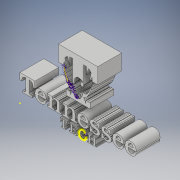
# Autodesk Inventor part: Main
Saved by Autodesk Inventor 2018 (Build 220112000, 112)
## iProperties
Created: 2017-12-08
Part Number: Main
Material: Generic
Document SubType Name: Modeling
Designer: Rus
Density: 1 g/cm^3
Appearance: Default
Author: Rus
Autodesk Inventor part; units mm, degrees
(part 1 of 3)
ref_plane "YZ Plane" through (0, 0, 0) normal (1, 0, 0) x (0, 1, 0)
ref_plane "XZ Plane" through (0, 0, 0) normal (0, 1, 0) x (-1, 0, 0)
ref_plane "XY Plane" through (0, 0, 0) normal (0, 0, 1) x (1, 0, 0)
sketch "Sketch1" plane through (0, 0, 0) normal (0, 0, 1) x (1, 0, 0)
  line L0 (63.7248, 41.0987) -> (64.7002, 37.0611)
  line L1 (64.7002, 37.0611) -> (64.5625, 36.9024)
  line L2 (64.5625, 36.9024) -> (63.8457, 36.2839)
  line L3 (63.8457, 36.2839) -> (63.0893, 35.88)
  line L4 (63.0893, 35.88) -> (62.9338, 35.8292)
  line L5 (62.9338, 35.8292) -> (61.9509, 40.717)
  line L6 (61.9509, 40.717) -> (61.0652, 35.7505)
  line L7 (61.0652, 35.7505) -> (60.894, 35.7889)
  line L8 (60.894, 35.7889) -> (60.0646, 36.1516)
  line L9 (60.0646, 36.1516) -> (59.2762, 36.7563)
  line L10 (59.2762, 36.7563) -> (59.1274, 36.9164)
  line L11 (59.1274, 36.9164) -> (60.1375, 41.0987)
  line L12 (60.1375, 41.0987) -> (58.1904, 38.2308)
  line L13 (58.1904, 38.2308) -> (58.0718, 38.4447)
  line L14 (58.0718, 38.4447) -> (57.5221, 39.6984)
  line L15 (57.5221, 39.6984) -> (57.0357, 41.2143)
  line L16 (57.0357, 41.2143) -> (56.9488, 41.5577)
  line L17 (56.9488, 41.5577) -> (55.9732, 44.7972)
  line L18 (55.9732, 44.7972) -> (55.9138, 44.5823)
  line L19 (55.9138, 44.5823) -> (55.6095, 43.9704)
  line L20 (55.6095, 43.9704) -> (55.1119, 43.5117)
  line L21 (55.1119, 43.5117) -> (54.5249, 43.3598)
  line L22 (54.5249, 43.3598) -> (53.8897, 43.4538)
  line L23 (53.8897, 43.4538) -> (53.2501, 43.7363)
  line L24 (53.2501, 43.7363) -> (52.6479, 44.1442)
  line L25 (52.6479, 44.1442) -> (52.1272, 44.6181)
  line L26 (52.1272, 44.6181) -> (51.8185, 44.971)
  line L27 (51.8185, 44.971) -> (51.7301, 45.0977)
  line L28 (51.7301, 45.0977) -> (51.1693, 45.9052)
  line L29 (51.1693, 45.9052) -> (49.7197, 48.4838)
  line L30 (49.7197, 48.4838) -> (48.2547, 51.9024)
  line L31 (48.2547, 51.9024) -> (47.3149, 55.134)
  line L32 (47.3149, 55.134) -> (46.9331, 57.2478)
  line L33 (46.9331, 57.2478) -> (46.8823, 57.9562)
  line L34 (46.8823, 57.9562) -> (46.8754, 57.8239)
  line L35 (46.8754, 57.8239) -> (46.845, 56.435)
  line L36 (46.845, 56.435) -> (46.8465, 56.2889)
  line L37 (46.8465, 56.2889) -> (46.8478, 55.5681)
  line L38 (46.8478, 55.5681) -> (47.147, 53.4045)
  line L39 (47.147, 53.4045) -> (48.0451, 49.9608)
  line L40 (48.0451, 49.9608) -> (49.5653, 46.2471)
  line L41 (49.5653, 46.2471) -> (51.1211, 43.4261)
  line L42 (51.1211, 43.4261) -> (51.7301, 42.5483)
  line L43 (51.7301, 42.5483) -> (51.8114, 42.431)
  line L44 (51.8114, 42.431) -> (52.0718, 42.0868)
  line L45 (52.0718, 42.0868) -> (52.528, 41.5369)
  line L46 (52.528, 41.5369) -> (53.0642, 40.9608)
  line L47 (53.0642, 40.9608) -> (53.6496, 40.4178)
  line L48 (53.6496, 40.4178) -> (54.2534, 39.973)
  line L49 (54.2534, 39.973) -> (54.8432, 39.686)
  line L50 (54.8432, 39.686) -> (55.3862, 39.6202)
  line L51 (55.3862, 39.6202) -> (55.7611, 39.7538)
  line L52 (55.7611, 39.7538) -> (55.8518, 39.8351)
  line L53 (55.8518, 39.8351) -> (55.8381, 39.7386)
  line L54 (55.8381, 39.7386) -> (55.5034, 38.7919)
  line L55 (55.5034, 38.7919) -> (55.4579, 38.7022)
  line L56 (55.4579, 38.7022) -> (53.5111, 34.8875)
  line L57 (53.5111, 34.8875) -> (53.5111, 38.0188)
  line L58 (53.5111, 38.0188) -> (53.4367, 38.0074)
  line L59 (53.4367, 38.0074) -> (52.6454, 37.9068)
  line L60 (52.6454, 37.9068) -> (52.5614, 37.8986)
  line L61 (52.5614, 37.8986) -> (52.3178, 37.875)
  line L62 (52.3178, 37.875) -> (50.9673, 37.7938)
  line L63 (50.9673, 37.7938) -> (49.567, 37.7592)
  line L64 (49.567, 37.7592) -> (49.1014, 37.7592)
  line L65 (49.1014, 37.7592) -> (49.1014, 32.2513)
  line L66 (49.1014, 32.2513) -> (74.6006, 32.2513)
  line L67 (74.6006, 32.2513) -> (74.6006, 37.7595)
  line L68 (74.6006, 37.7595) -> (74.1252, 37.7704)
  line L69 (74.1252, 37.7704) -> (72.1808, 37.841)
  line L70 (72.1808, 37.841) -> (70.8138, 37.9317)
  line L71 (70.8138, 37.9317) -> (70.6278, 37.9523)
  line L72 (70.6278, 37.9523) -> (70.5933, 37.9566)
  line L73 (70.5933, 37.9566) -> (70.2641, 37.9952)
  line L74 (70.2641, 37.9952) -> (70.2323, 37.9993)
  line L75 (70.2323, 37.9993) -> (70.2323, 34.8875)
  line L76 (70.2323, 34.8875) -> (68.2214, 38.8246)
  line L77 (68.2214, 38.8246) -> (68.1802, 38.9059)
  line L78 (68.1802, 38.9059) -> (67.9361, 39.6747)
  line L79 (67.9361, 39.6747) -> (67.9236, 39.7672)
  line L80 (67.9236, 39.7672) -> (68.0189, 39.6996)
  line L81 (68.0189, 39.6996) -> (68.3935, 39.6143)
  line L82 (68.3935, 39.6143) -> (68.9323, 39.7175)
  line L83 (68.9323, 39.7175) -> (69.5098, 40.0208)
  line L84 (69.5098, 40.0208) -> (70.0981, 40.4687)
  line L85 (70.0981, 40.4687) -> (70.6662, 41.0034)
  line L86 (70.6662, 41.0034) -> (71.1853, 41.5655)
  line L87 (71.1853, 41.5655) -> (71.6262, 42.1005)
  line L88 (71.6262, 42.1005) -> (71.88, 42.434)
  line L89 (71.88, 42.434) -> (71.9597, 42.5483)
  line L90 (71.9597, 42.5483) -> (72.5675, 43.4261)
  line L91 (72.5675, 43.4261) -> (74.1218, 46.2471)
  line L92 (74.1218, 46.2471) -> (75.642, 49.9608)
  line L93 (75.642, 49.9608) -> (76.5419, 53.4045)
  line L94 (76.5419, 53.4045) -> (76.8406, 55.5681)
  line L95 (76.8406, 55.5681) -> (76.8434, 56.2889)
  line L96 (76.8434, 56.2889) -> (76.8434, 56.435)
  line L97 (76.8434, 56.435) -> (76.8132, 57.8239)
  line L98 (76.8132, 57.8239) -> (76.8078, 57.9562)
  line L99 (76.8078, 57.9562) -> (76.7552, 57.2463)
  line L100 (76.7552, 57.2463) -> (76.3735, 55.134)
  line L101 (76.3735, 55.134) -> (75.4337, 51.9024)
  line L102 (75.4337, 51.9024) -> (73.9676, 48.4838)
  line L103 (73.9676, 48.4838) -> (72.519, 45.9039)
  line L104 (72.519, 45.9039) -> (71.9597, 45.0977)
  line L105 (71.9597, 45.0977) -> (71.8703, 44.971)
  line L106 (71.8703, 44.971) -> (71.5617, 44.6181)
  line L107 (71.5617, 44.6181) -> (71.0408, 44.1442)
  line L108 (71.0408, 44.1442) -> (70.4385, 43.7363)
  line L109 (70.4385, 43.7363) -> (69.7989, 43.4538)
  line L110 (69.7989, 43.4538) -> (69.1639, 43.3598)
  line L111 (69.1639, 43.3598) -> (68.5754, 43.5117)
  line L112 (68.5754, 43.5117) -> (68.0791, 43.9704)
  line L113 (68.0791, 43.9704) -> (67.7746, 44.5823)
  line L114 (67.7746, 44.5823) -> (67.7167, 44.7972)
  line L115 (67.7167, 44.7972) -> (66.74, 41.5577)
  line L116 (66.74, 41.5577) -> (66.657, 41.2323)
  line L117 (66.657, 41.2323) -> (66.2008, 39.7881)
  line L118 (66.2008, 39.7881) -> (65.6869, 38.578)
  line L119 (65.6869, 38.578) -> (65.5767, 38.3703)
  line L120 (65.5767, 38.3703) -> (63.7248, 41.0987)
  line L121 (82.8011, 75.2394) -> (82.8011, 58.6456)
  line L122 (82.8011, 58.6456) -> (76.9705, 58.6456)
  line L123 (76.9705, 58.6456) -> (76.9705, 59.5536)
  line L124 (76.9705, 59.5536) -> (76.7432, 62.0052)
  line L125 (76.7432, 62.0052) -> (76.6974, 62.2752)
  line L126 (76.6974, 62.2752) -> (73.8313, 57.2978)
  line L127 (73.8313, 57.2978) -> (75.8254, 65.5592)
  line L128 (75.8254, 65.5592) -> (75.6723, 65.9148)
  line L129 (75.6723, 65.9148) -> (74.6885, 67.3796)
  line L130 (74.6885, 67.3796) -> (73.3972, 68.4558)
  line L131 (73.3972, 68.4558) -> (73.0924, 68.6156)
  line L132 (73.0924, 68.6156) -> (70.874, 61.7462)
  line L133 (70.874, 61.7462) -> (70.7833, 69.3639)
  line L134 (70.7833, 69.3639) -> (70.5542, 69.4037)
  line L135 (70.5542, 69.4037) -> (67.9857, 69.546)
  line L136 (67.9857, 69.546) -> (67.7002, 69.5346)
  line L137 (67.7002, 69.5346) -> (67.7117, 50.8236)
  line L138 (67.7117, 50.8236) -> (67.7117, 50.544)
  line L139 (67.7117, 50.544) -> (67.4744, 49.7022)
  line L140 (67.4744, 49.7022) -> (66.8609, 48.954)
  line L141 (66.8609, 48.954) -> (66.023, 48.6754)
  line L142 (66.023, 48.6754) -> (65.3008, 48.8355)
  line L143 (65.3008, 48.8355) -> (65.1109, 48.9623)
  line L144 (65.1109, 48.9623) -> (64.9321, 49.0822)
  line L145 (64.9321, 49.0822) -> (64.5267, 49.6308)
  line L146 (64.5267, 49.6308) -> (64.2924, 50.529)
  line L147 (64.2924, 50.529) -> (64.4718, 51.4815)
  line L148 (64.4718, 51.4815) -> (64.928, 52.1525)
  line L149 (64.928, 52.1525) -> (65.132, 52.3067)
  line L150 (65.132, 52.3067) -> (66.0855, 52.4872)
  line L151 (66.0855, 52.4872) -> (66.6036, 52.1895)
  line L152 (66.6036, 52.1895) -> (66.6369, 52.432)
  line L153 (66.6369, 52.432) -> (66.5816, 53.1803)
  line L154 (66.5816, 53.1803) -> (66.2235, 53.8128)
  line L155 (66.2235, 53.8128) -> (65.5952, 54.1575)
  line L156 (65.5952, 54.1575) -> (64.9693, 54.2719)
  line L157 (64.9693, 54.2719) -> (64.7598, 54.2788)
  line L158 (64.7598, 54.2788) -> (64.4337, 54.4825)
  line L159 (64.4337, 54.4825) -> (63.3298, 54.8895)
  line L160 (63.3298, 54.8895) -> (61.9572, 54.9707)
  line L161 (61.9572, 54.9707) -> (60.6991, 54.592)
  line L162 (60.6991, 54.592) -> (59.6089, 53.8215)
  line L163 (59.6089, 53.8215) -> (58.7472, 52.7319)
  line L164 (58.7472, 52.7319) -> (58.1687, 51.3896)
  line L165 (58.1687, 51.3896) -> (57.9301, 49.8656)
  line L166 (57.9301, 49.8656) -> (57.9988, 48.6253)
  line L167 (57.9988, 48.6253) -> (58.0882, 48.2255)
  line L168 (58.0882, 48.2255) -> (58.1258, 48.0576)
  line L169 (58.1258, 48.0576) -> (58.1006, 47.4831)
  line L170 (58.1006, 47.4831) -> (57.7932, 47.1882)
  line L171 (57.7932, 47.1882) -> (57.6898, 47.1605)
  line L172 (57.6898, 47.1605) -> (57.5163, 47.1151)
  line L173 (57.5163, 47.1151) -> (56.9388, 47.1852)
  line L174 (56.9388, 47.1852) -> (56.4031, 47.6234)
  line L175 (56.4031, 47.6234) -> (56.0821, 48.3415)
  line L176 (56.0821, 48.3415) -> (55.976, 48.9892)
  line L177 (55.976, 48.9892) -> (55.976, 49.2044)
  line L178 (55.976, 49.2044) -> (55.9897, 69.5355)
  line L179 (55.9897, 69.5355) -> (55.703, 69.547)
  line L180 (55.703, 69.547) -> (53.1343, 69.4047)
  line L181 (53.1343, 69.4047) -> (52.9072, 69.3649)
  line L182 (52.9072, 69.3649) -> (52.816, 61.7471)
  line L183 (52.816, 61.7471) -> (50.5976, 68.6166)
  line L184 (50.5976, 68.6166) -> (50.2917, 68.4568)
  line L185 (50.2917, 68.4568) -> (49.0014, 67.3791)
  line L186 (49.0014, 67.3791) -> (48.0162, 65.9145)
  line L187 (48.0162, 65.9145) -> (47.8648, 65.5602)
  line L188 (47.8648, 65.5602) -> (49.8574, 57.2988)
  line L189 (49.8574, 57.2988) -> (47.0063, 62.2529)
  line L190 (47.0063, 62.2529) -> (46.9593, 61.9841)
  line L191 (46.9593, 61.9841) -> (46.7307, 59.4815)
  line L192 (46.7307, 59.4815) -> (46.7307, 58.6466)
  line L193 (46.7307, 58.6466) -> (40.9636, 58.6466)
  line L194 (40.9636, 58.6466) -> (40.9636, 75.2394)
  line L195 (40.9636, 75.2394) -> (82.8011, 75.2394)
  line L196 (6.1983, 26.6612) -> (5.8648, 26.6612)
  line L197 (5.8648, 26.6612) -> (5.4238, 26.6612)
  line L198 (5.4238, 26.6612) -> (4.1051, 26.3565)
  line L199 (4.1051, 26.3565) -> (3.0565, 25.6467)
  line L200 (3.0565, 25.6467) -> (2.9022, 25.4442)
  line L201 (2.9022, 25.4442) -> (2.7478, 25.2415)
  line L202 (2.7478, 25.2415) -> (2.198, 23.8497)
  line L203 (2.198, 23.8497) -> (1.9444, 21.9535)
  line L204 (1.9444, 21.9535) -> (1.9389, 21.4988)
  line L205 (1.9389, 21.4988) -> (0, 21.4988)
  line L206 (0, 21.4988) -> (0, 28.5255)
  line L207 (0, 28.5255) -> (15.9768, 28.5255)
  line L208 (15.9768, 28.5255) -> (15.9768, 21.4991)
  line L209 (15.9768, 21.4991) -> (14.0379, 21.4991)
  line L210 (14.0379, 21.4991) -> (14.0338, 21.9483)
  line L211 (14.0338, 21.9483) -> (13.7871, 23.828)
  line L212 (13.7871, 23.828) -> (13.2414, 25.2212)
  line L213 (13.2414, 25.2212) -> (13.0871, 25.4265)
  line L214 (13.0871, 25.4265) -> (12.9327, 25.6333)
  line L215 (12.9327, 25.6333) -> (11.8854, 26.3526)
  line L216 (11.8854, 26.3526) -> (10.5736, 26.6612)
  line L217 (10.5736, 26.6612) -> (10.1367, 26.6612)
  line L218 (10.1367, 26.6612) -> (9.766, 26.6612)
  line L219 (9.766, 26.6612) -> (9.766, 15.0554)
  line L220 (9.766, 15.0554) -> (9.766, 14.8473)
  line L221 (9.766, 14.8473) -> (9.8349, 14.2189)
  line L222 (9.8349, 14.2189) -> (9.9975, 13.8041)
  line L223 (9.9975, 13.8041) -> (10.0444, 13.7587)
  line L224 (10.0444, 13.7587) -> (10.0898, 13.7132)
  line L225 (10.0898, 13.7132) -> (10.5363, 13.5547)
  line L226 (10.5363, 13.5547) -> (11.2267, 13.4872)
  line L227 (11.2267, 13.4872) -> (11.4582, 13.4872)
  line L228 (11.4582, 13.4872) -> (12.9024, 13.4872)
  line L229 (12.9024, 13.4872) -> (12.9024, 11.5607)
  line L230 (12.9024, 11.5607) -> (3.0618, 11.5607)
  line L231 (3.0618, 11.5607) -> (3.0618, 13.4872)
  line L232 (3.0618, 13.4872) -> (4.5308, 13.4872)
  line L233 (4.5308, 13.4872) -> (4.7582, 13.4872)
  line L234 (4.7582, 13.4872) -> (5.4417, 13.5533)
  line L235 (5.4417, 13.5533) -> (5.8813, 13.7077)
  line L236 (5.8813, 13.7077) -> (5.9268, 13.7518)
  line L237 (5.9268, 13.7518) -> (5.9709, 13.7973)
  line L238 (5.9709, 13.7973) -> (6.1293, 14.2121)
  line L239 (6.1293, 14.2121) -> (6.1983, 14.8446)
  line L240 (6.1983, 14.8446) -> (6.1983, 15.0554)
  line L241 (6.1983, 15.0554) -> (6.1983, 26.6612)
  line L242 (24.6021, 19.0679) -> (24.5828, 19.3435)
  line L243 (24.5828, 19.3435) -> (24.3775, 20.4997)
  line L244 (24.3775, 20.4997) -> (24.022, 21.3596)
  line L245 (24.022, 21.3596) -> (23.9282, 21.4864)
  line L246 (23.9282, 21.4864) -> (23.8345, 21.6145)
  line L247 (23.8345, 21.6145) -> (23.2351, 22.0624)
  line L248 (23.2351, 22.0624) -> (22.5185, 22.2526)
  line L249 (22.5185, 22.2526) -> (22.2801, 22.2526)
  line L250 (22.2801, 22.2526) -> (22.0279, 22.2526)
  line L251 (22.0279, 22.2526) -> (21.2728, 22.0514)
  line L252 (21.2728, 22.0514) -> (20.5879, 21.5787)
  line L253 (20.5879, 21.5787) -> (20.4721, 21.4437)
  line L254 (20.4721, 21.4437) -> (20.355, 21.31)
  line L255 (20.355, 21.31) -> (19.892, 20.4459)
  line L256 (19.892, 20.4459) -> (19.5888, 19.3298)
  line L257 (19.5888, 19.3298) -> (19.5516, 19.0679)
  line L258 (19.5516, 19.0679) -> (24.6021, 19.0679)
  line L259 (25.7492, 15.8331) -> (27.8727, 15.8331)
  line L260 (27.8727, 15.8331) -> (27.8273, 15.4679)
  line L261 (27.8273, 15.4679) -> (27.2972, 13.8693)
  line L262 (27.2972, 13.8693) -> (26.3617, 12.5807)
  line L263 (26.3617, 12.5807) -> (26.1135, 12.3698)
  line L264 (26.1135, 12.3698) -> (25.8657, 12.1589)
  line L265 (25.8657, 12.1589) -> (24.4174, 11.4214)
  line L266 (24.4174, 11.4214) -> (22.8327, 11.1042)
  line L267 (22.8327, 11.1042) -> (22.3049, 11.1042)
  line L268 (22.3049, 11.1042) -> (21.9618, 11.1042)
  line L269 (21.9618, 11.1042) -> (20.9338, 11.2145)
  line L270 (20.9338, 11.2145) -> (19.7087, 11.541)
  line L271 (19.7087, 11.541) -> (18.6297, 12.0868)
  line L272 (18.6297, 12.0868) -> (17.909, 12.638)
  line L273 (17.909, 12.638) -> (17.6995, 12.8502)
  line L274 (17.6995, 12.8502) -> (17.4887, 13.0652)
  line L275 (17.4887, 13.0652) -> (16.9485, 13.7983)
  line L276 (16.9485, 13.7983) -> (16.4124, 14.8925)
  line L277 (16.4124, 14.8925) -> (16.09, 16.1355)
  line L278 (16.09, 16.1355) -> (15.9839, 17.1772)
  line L279 (15.9839, 17.1772) -> (15.9839, 17.5245)
  line L280 (15.9839, 17.5245) -> (15.9839, 17.869)
  line L281 (15.9839, 17.869) -> (16.0914, 18.8998)
  line L282 (16.0914, 18.8998) -> (16.4166, 20.1345)
  line L283 (16.4166, 20.1345) -> (16.9581, 21.2301)
  line L284 (16.9581, 21.2301) -> (17.5066, 21.9687)
  line L285 (17.5066, 21.9687) -> (17.7188, 22.185)
  line L286 (17.7188, 22.185) -> (17.9297, 22.4014)
  line L287 (17.9297, 22.4014) -> (18.6545, 22.9609)
  line L288 (18.6545, 22.9609) -> (19.7321, 23.5134)
  line L289 (19.7321, 23.5134) -> (20.9476, 23.8456)
  line L290 (20.9476, 23.8456) -> (21.9645, 23.9558)
  line L291 (21.9645, 23.9558) -> (22.3049, 23.9558)
  line L292 (22.3049, 23.9558) -> (22.6274, 23.9558)
  line L293 (22.6274, 23.9558) -> (23.5989, 23.8497)
  line L294 (23.5989, 23.8497) -> (24.7303, 23.53)
  line L295 (24.7303, 23.53) -> (25.699, 22.9953)
  line L296 (25.699, 22.9953) -> (26.3273, 22.4551)
  line L297 (26.3273, 22.4551) -> (26.5039, 22.247)
  line L298 (26.5039, 22.247) -> (26.6857, 22.0307)
  line L299 (26.6857, 22.0307) -> (27.1351, 21.2948)
  line L300 (27.1351, 21.2948) -> (27.5856, 20.1496)
  line L301 (27.5856, 20.1496) -> (27.8569, 18.8102)
  line L302 (27.8569, 18.8102) -> (27.9479, 17.6601)
  line L303 (27.9479, 17.6601) -> (27.9479, 17.2771)
  line L304 (27.9479, 17.2771) -> (19.4279, 17.2771)
  line L305 (19.4279, 17.2771) -> (19.4389, 16.9409)
  line L306 (19.4389, 16.9409) -> (19.6789, 15.494)
  line L307 (19.6789, 15.494) -> (20.1544, 14.3682)
  line L308 (20.1544, 14.3682) -> (20.2853, 14.1904)
  line L309 (20.2853, 14.1904) -> (20.4162, 14.014)
  line L310 (20.4162, 14.014) -> (21.228, 13.3954)
  line L311 (21.228, 13.3954) -> (22.1747, 13.1294)
  line L312 (22.1747, 13.1294) -> (22.4902, 13.1294)
  line L313 (22.4902, 13.1294) -> (22.8086, 13.1294)
  line L314 (22.8086, 13.1294) -> (23.7677, 13.2865)
  line L315 (23.7677, 13.2865) -> (24.5684, 13.6489)
  line L316 (24.5684, 13.6489) -> (24.6937, 13.7522)
  line L317 (24.6937, 13.7522) -> (24.8178, 13.8569)
  line L318 (24.8178, 13.8569) -> (25.3304, 14.5846)
  line L319 (25.3304, 14.5846) -> (25.6969, 15.5906)
  line L320 (25.6969, 15.5906) -> (25.7492, 15.8331)
  line L321 (28.9885, 11.5604) -> (28.9885, 13.2512)
  line L322 (28.9885, 13.2512) -> (29.829, 13.2512)
  line L323 (29.829, 13.2512) -> (30.0081, 13.2512)
  line L324 (30.0081, 13.2512) -> (30.5471, 13.3201)
  line L325 (30.5471, 13.3201) -> (30.9288, 13.4786)
  line L326 (30.9288, 13.4786) -> (30.9768, 13.5227)
  line L327 (30.9768, 13.5227) -> (31.0238, 13.5681)
  line L328 (31.0238, 13.5681) -> (31.1892, 13.9719)
  line L329 (31.1892, 13.9719) -> (31.2608, 14.5714)
  line L330 (31.2608, 14.5714) -> (31.2608, 14.7698)
  line L331 (31.2608, 14.7698) -> (31.2608, 20.2889)
  line L332 (31.2608, 20.2889) -> (31.2608, 20.4887)
  line L333 (31.2608, 20.4887) -> (31.1892, 21.0881)
  line L334 (31.1892, 21.0881) -> (31.0238, 21.4864)
  line L335 (31.0238, 21.4864) -> (30.9768, 21.5305)
  line L336 (30.9768, 21.5305) -> (30.9288, 21.5746)
  line L337 (30.9288, 21.5746) -> (30.5471, 21.7303)
  line L338 (30.5471, 21.7303) -> (30.0081, 21.7965)
  line L339 (30.0081, 21.7965) -> (29.829, 21.7965)
  line L340 (29.829, 21.7965) -> (28.9885, 21.7965)
  line L341 (28.9885, 21.7965) -> (28.9885, 23.4997)
  line L342 (28.9885, 23.4997) -> (34.3228, 23.4997)
  line L343 (34.3228, 23.4997) -> (34.3228, 21.401)
  line L344 (34.3228, 21.401) -> (34.4869, 21.6077)
  line L345 (34.4869, 21.6077) -> (36.1793, 23.1511)
  line L346 (36.1793, 23.1511) -> (36.354, 23.2531)
  line L347 (36.354, 23.2531) -> (36.5278, 23.3564)
  line L348 (36.5278, 23.3564) -> (37.9842, 23.8704)
  line L349 (37.9842, 23.8704) -> (38.4709, 23.8704)
  line L350 (38.4709, 23.8704) -> (38.9131, 23.8704)
  line L351 (38.9131, 23.8704) -> (40.2428, 23.6182)
  line L352 (40.2428, 23.6182) -> (41.2847, 23.0271)
  line L353 (41.2847, 23.0271) -> (41.4348, 22.8576)
  line L354 (41.4348, 22.8576) -> (41.5852, 22.6894)
  line L355 (41.5852, 22.6894) -> (42.1099, 21.5057)
  line L356 (42.1099, 21.5057) -> (42.3362, 19.983)
  line L357 (42.3362, 19.983) -> (42.3362, 19.4745)
  line L358 (42.3362, 19.4745) -> (42.3362, 14.7699)
  line L359 (42.3362, 14.7699) -> (42.3362, 14.5714)
  line L360 (42.3362, 14.5714) -> (42.4079, 13.972)
  line L361 (42.4079, 13.972) -> (42.577, 13.5682)
  line L362 (42.577, 13.5682) -> (42.6255, 13.5227)
  line L363 (42.6255, 13.5227) -> (42.6738, 13.4786)
  line L364 (42.6738, 13.4786) -> (43.0596, 13.3202)
  line L365 (43.0596, 13.3202) -> (43.5999, 13.2512)
  line L366 (43.5999, 13.2512) -> (43.7805, 13.2512)
  line L367 (43.7805, 13.2512) -> (44.5216, 13.2512)
  line L368 (44.5216, 13.2512) -> (44.5216, 11.5604)
  line L369 (44.5216, 11.5604) -> (37.3352, 11.5604)
  line L370 (37.3352, 11.5604) -> (37.3352, 13.2512)
  line L371 (37.3352, 13.2512) -> (37.8424, 13.2512)
  line L372 (37.8424, 13.2512) -> (38.0213, 13.2512)
  line L373 (38.0213, 13.2512) -> (38.5618, 13.3201)
  line L374 (38.5618, 13.3201) -> (38.9473, 13.4786)
  line L375 (38.9473, 13.4786) -> (38.9956, 13.5227)
  line L376 (38.9956, 13.5227) -> (39.0441, 13.5681)
  line L377 (39.0441, 13.5681) -> (39.2133, 13.9719)
  line L378 (39.2133, 13.9719) -> (39.2864, 14.5714)
  line L379 (39.2864, 14.5714) -> (39.2864, 14.7698)
  line L380 (39.2864, 14.7698) -> (39.2864, 19.4744)
  line L381 (39.2864, 19.4744) -> (39.2864, 19.7583)
  line L382 (39.2864, 19.7583) -> (39.1765, 20.6072)
  line L383 (39.1765, 20.6072) -> (38.9212, 21.27)
  line L384 (38.9212, 21.27) -> (38.8483, 21.3637)
  line L385 (38.8483, 21.3637) -> (38.7739, 21.4588)
  line L386 (38.7739, 21.4588) -> (38.2681, 21.7909)
  line L387 (38.2681, 21.7909) -> (37.623, 21.9315)
  line L388 (37.623, 21.9315) -> (37.4096, 21.9315)
  line L389 (37.4096, 21.9315) -> (37.0886, 21.9315)
  line L390 (37.0886, 21.9315) -> (36.1279, 21.66)
  line L391 (36.1279, 21.66) -> (35.2872, 21.0275)
  line L392 (35.2872, 21.0275) -> (35.1495, 20.8456)
  line L393 (35.1495, 20.8456) -> (35.0119, 20.6651)
  line L394 (35.0119, 20.6651) -> (34.5295, 19.5557)
  line L395 (34.5295, 19.5557) -> (34.3228, 18.2824)
  line L396 (34.3228, 18.2824) -> (34.3228, 17.8566)
  line L397 (34.3228, 17.8566) -> (34.3228, 14.7698)
  line L398 (34.3228, 14.7698) -> (34.3228, 14.5714)
  line L399 (34.3228, 14.5714) -> (34.3944, 13.9719)
  line L400 (34.3944, 13.9719) -> (34.5641, 13.5681)
  line L401 (34.5641, 13.5681) -> (34.6121, 13.5227)
  line L402 (34.6121, 13.5227) -> (34.6603, 13.4786)
  line L403 (34.6603, 13.4786) -> (35.0464, 13.3201)
  line L404 (35.0464, 13.3201) -> (35.5864, 13.2512)
  line L405 (35.5864, 13.2512) -> (35.767, 13.2512)
  line L406 (35.767, 13.2512) -> (36.274, 13.2512)
  line L407 (36.274, 13.2512) -> (36.274, 11.5604)
  line L408 (36.274, 11.5604) -> (28.9885, 11.5604)
  line L409 (45.3182, 11.5604) -> (45.3182, 13.2512)
  line L410 (45.3182, 13.2512) -> (46.1574, 13.2512)
  line L411 (46.1574, 13.2512) -> (46.3367, 13.2512)
  line L412 (46.3367, 13.2512) -> (46.8767, 13.3201)
  line L413 (46.8767, 13.3201) -> (47.2585, 13.4786)
  line L414 (47.2585, 13.4786) -> (47.3067, 13.5227)
  line L415 (47.3067, 13.5227) -> (47.3535, 13.5681)
  line L416 (47.3535, 13.5681) -> (47.5188, 13.9719)
  line L417 (47.5188, 13.9719) -> (47.5905, 14.5714)
  line L418 (47.5905, 14.5714) -> (47.5905, 14.7698)
  line L419 (47.5905, 14.7698) -> (47.5905, 20.2889)
  line L420 (47.5905, 20.2889) -> (47.5905, 20.4887)
  line L421 (47.5905, 20.4887) -> (47.5188, 21.0881)
  line L422 (47.5188, 21.0881) -> (47.3535, 21.4864)
  line L423 (47.3535, 21.4864) -> (47.3068, 21.5305)
  line L424 (47.3068, 21.5305) -> (47.2585, 21.5746)
  line L425 (47.2585, 21.5746) -> (46.8767, 21.7303)
  line L426 (46.8767, 21.7303) -> (46.3367, 21.7965)
  line L427 (46.3367, 21.7965) -> (46.1574, 21.7965)
  line L428 (46.1574, 21.7965) -> (45.3182, 21.7965)
  line L429 (45.3182, 21.7965) -> (45.3182, 23.4997)
  line L430 (45.3182, 23.4997) -> (50.6525, 23.4997)
  line L431 (50.6525, 23.4997) -> (50.6525, 21.401)
  line L432 (50.6525, 21.401) -> (50.8165, 21.6077)
  line L433 (50.8165, 21.6077) -> (52.5089, 23.1511)
  line L434 (52.5089, 23.1511) -> (52.6839, 23.2531)
  line L435 (52.6839, 23.2531) -> (52.8574, 23.3564)
  line L436 (52.8574, 23.3564) -> (54.3141, 23.8705)
  line L437 (54.3141, 23.8705) -> (54.8005, 23.8705)
  line L438 (54.8005, 23.8705) -> (55.243, 23.8705)
  line L439 (55.243, 23.8705) -> (56.5711, 23.6183)
  line L440 (56.5711, 23.6183) -> (57.6133, 23.0271)
  line L441 (57.6133, 23.0271) -> (57.7632, 22.8577)
  line L442 (57.7632, 22.8577) -> (57.9135, 22.6895)
  line L443 (57.9135, 22.6895) -> (58.4398, 21.5058)
  line L444 (58.4398, 21.5058) -> (58.6659, 19.983)
  line L445 (58.6659, 19.983) -> (58.6659, 19.4746)
  line L446 (58.6659, 19.4746) -> (58.6659, 14.7699)
  line L447 (58.6659, 14.7699) -> (58.6659, 14.5715)
  line L448 (58.6659, 14.5715) -> (58.7375, 13.9721)
  line L449 (58.7375, 13.9721) -> (58.9069, 13.5683)
  line L450 (58.9069, 13.5683) -> (58.9552, 13.5228)
  line L451 (58.9552, 13.5228) -> (59.0034, 13.4787)
  line L452 (59.0034, 13.4787) -> (59.388, 13.3202)
  line L453 (59.388, 13.3202) -> (59.9295, 13.2513)
  line L454 (59.9295, 13.2513) -> (60.1101, 13.2513)
  line L455 (60.1101, 13.2513) -> (60.8501, 13.2513)
  line L456 (60.8501, 13.2513) -> (60.8501, 11.5604)
  line L457 (60.8501, 11.5604) -> (53.6649, 11.5604)
  line L458 (53.6649, 11.5604) -> (53.6649, 13.2513)
  line L459 (53.6649, 13.2513) -> (54.1709, 13.2513)
  line L460 (54.1709, 13.2513) -> (54.35, 13.2513)
  line L461 (54.35, 13.2513) -> (54.8915, 13.3202)
  line L462 (54.8915, 13.3202) -> (55.2771, 13.4787)
  line L463 (55.2771, 13.4787) -> (55.3256, 13.5228)
  line L464 (55.3256, 13.5228) -> (55.3738, 13.5682)
  line L465 (55.3738, 13.5682) -> (55.5433, 13.972)
  line L466 (55.5433, 13.972) -> (55.6162, 14.5715)
  line L467 (55.6162, 14.5715) -> (55.6162, 14.7699)
  line L468 (55.6162, 14.7699) -> (55.6162, 19.4745)
  line L469 (55.6162, 19.4745) -> (55.6162, 19.7584)
  line L470 (55.6162, 19.7584) -> (55.5062, 20.6073)
  line L471 (55.5062, 20.6073) -> (55.2496, 21.2701)
  line L472 (55.2496, 21.2701) -> (55.1767, 21.3638)
  line L473 (55.1767, 21.3638) -> (55.1036, 21.4589)
  line L474 (55.1036, 21.4589) -> (54.5981, 21.791)
  line L475 (54.5981, 21.791) -> (53.9532, 21.9315)
  line L476 (53.9532, 21.9315) -> (53.7393, 21.9315)
  line L477 (53.7393, 21.9315) -> (53.4182, 21.9315)
  line L478 (53.4182, 21.9315) -> (52.4576, 21.66)
  line L479 (52.4576, 21.66) -> (51.6171, 21.0275)
  line L480 (51.6171, 21.0275) -> (51.4795, 20.8456)
  line L481 (51.4795, 20.8456) -> (51.3415, 20.6651)
  line L482 (51.3415, 20.6651) -> (50.8592, 19.5557)
  line L483 (50.8592, 19.5557) -> (50.6524, 18.2824)
  line L484 (50.6524, 18.2824) -> (50.6524, 17.8566)
  line L485 (50.6524, 17.8566) -> (50.6524, 14.7698)
  line L486 (50.6524, 14.7698) -> (50.6524, 14.5714)
  line L487 (50.6524, 14.5714) -> (50.7241, 13.9719)
  line L488 (50.7241, 13.9719) -> (50.8937, 13.5681)
  line L489 (50.8937, 13.5681) -> (50.9417, 13.5227)
  line L490 (50.9417, 13.5227) -> (50.9902, 13.4786)
  line L491 (50.9902, 13.4786) -> (51.3761, 13.3201)
  line L492 (51.3761, 13.3201) -> (51.9161, 13.2512)
  line L493 (51.9161, 13.2512) -> (52.0969, 13.2512)
  line L494 (52.0969, 13.2512) -> (52.6024, 13.2512)
  line L495 (52.6024, 13.2512) -> (52.6024, 11.5604)
  line L496 (52.6024, 11.5604) -> (45.3182, 11.5604)
  line L497 (69.6557, 19.0679) -> (69.6366, 19.3435)
  line L498 (69.6366, 19.3435) -> (69.4324, 20.4997)
  line L499 (69.4324, 20.4997) -> (69.0771, 21.3596)
  line L500 (69.0771, 21.3596) -> (68.9834, 21.4864)
  line L501 (68.9834, 21.4864) -> (68.8894, 21.6145)
  line L502 (68.8894, 21.6145) -> (68.2899, 22.0624)
  line L503 (68.2899, 22.0624) -> (67.5734, 22.2526)
  line L504 (67.5734, 22.2526) -> (67.3351, 22.2526)
  line L505 (67.3351, 22.2526) -> (67.0829, 22.2526)
  line L506 (67.0829, 22.2526) -> (66.3265, 22.0514)
  line L507 (66.3265, 22.0514) -> (65.6415, 21.5787)
  line L508 (65.6415, 21.5787) -> (65.5256, 21.4437)
  line L509 (65.5256, 21.4437) -> (65.4086, 21.31)
  line L510 (65.4086, 21.31) -> (64.947, 20.4459)
  line L511 (64.947, 20.4459) -> (64.6422, 19.3298)
  line L512 (64.6422, 19.3298) -> (64.6067, 19.0679)
  line L513 (64.6067, 19.0679) -> (69.6557, 19.0679)
  line L514 (70.8029, 15.8326) -> (72.9281, 15.8326)
  line L515 (72.9281, 15.8326) -> (72.8827, 15.4674)
  line L516 (72.8827, 15.4674) -> (72.3522, 13.8688)
  line L517 (72.3522, 13.8688) -> (71.4164, 12.5803)
  line L518 (71.4164, 12.5803) -> (71.1685, 12.3694)
  line L519 (71.1685, 12.3694) -> (70.9204, 12.1585)
  line L520 (70.9204, 12.1585) -> (69.4724, 11.4212)
  line L521 (69.4724, 11.4212) -> (67.8877, 11.104)
  line L522 (67.8877, 11.104) -> (67.3597, 11.104)
  line L523 (67.3597, 11.104) -> (67.0168, 11.104)
  line L524 (67.0168, 11.104) -> (65.9873, 11.2143)
  line L525 (65.9873, 11.2143) -> (64.7636, 11.541)
  line L526 (64.7636, 11.541) -> (63.6844, 12.0868)
  line L527 (63.6844, 12.0868) -> (62.9637, 12.6379)
  line L528 (62.9637, 12.6379) -> (62.7544, 12.8502)
  line L529 (62.7544, 12.8502) -> (62.5436, 13.0651)
  line L530 (62.5436, 13.0651) -> (62.0034, 13.7983)
  line L531 (62.0034, 13.7983) -> (61.4673, 14.8925)
  line L532 (61.4673, 14.8925) -> (61.1449, 16.1354)
  line L533 (61.1449, 16.1354) -> (61.0387, 17.1772)
  line L534 (61.0387, 17.1772) -> (61.0387, 17.5245)
  line L535 (61.0387, 17.5245) -> (61.0387, 17.869)
  line L536 (61.0387, 17.869) -> (61.1462, 18.8998)
  line L537 (61.1462, 18.8998) -> (61.4717, 20.1345)
  line L538 (61.4717, 20.1345) -> (62.0132, 21.23)
  line L539 (62.0132, 21.23) -> (62.5603, 21.9686)
  line L540 (62.5603, 21.9686) -> (62.7727, 22.185)
  line L541 (62.7727, 22.185) -> (62.9833, 22.4013)
  line L542 (62.9833, 22.4013) -> (63.7097, 22.9608)
  line L543 (63.7097, 22.9608) -> (64.7872, 23.5133)
  line L544 (64.7872, 23.5133) -> (66.0028, 23.8455)
  line L545 (66.0028, 23.8455) -> (67.0199, 23.9558)
  line L546 (67.0199, 23.9558) -> (67.36, 23.9558)
  line L547 (67.36, 23.9558) -> (67.6823, 23.9558)
  line L548 (67.6823, 23.9558) -> (68.6538, 23.8496)
  line L549 (68.6538, 23.8496) -> (69.7852, 23.5299)
  line L550 (69.7852, 23.5299) -> (70.7529, 22.9953)
  line L551 (70.7529, 22.9953) -> (71.3813, 22.4551)
  line L552 (71.3813, 22.4551) -> (71.5576, 22.247)
  line L553 (71.5576, 22.247) -> (71.7392, 22.0306)
  line L554 (71.7392, 22.0306) -> (72.1888, 21.2948)
  line L555 (72.1888, 21.2948) -> (72.6406, 20.1496)
  line L556 (72.6406, 20.1496) -> (72.9124, 18.8102)
  line L557 (72.9124, 18.8102) -> (73.0028, 17.6601)
  line L558 (73.0028, 17.6601) -> (73.0028, 17.2768)
  line L559 (73.0028, 17.2768) -> (64.4819, 17.2768)
  line L560 (64.4819, 17.2768) -> (64.4943, 16.9406)
  line L561 (64.4943, 16.9406) -> (64.7328, 15.4936)
  line L562 (64.7328, 15.4936) -> (65.2095, 14.3678)
  line L563 (65.2095, 14.3678) -> (65.3405, 14.19)
  line L564 (65.3405, 14.19) -> (65.4698, 14.0136)
  line L565 (65.4698, 14.0136) -> (66.2832, 13.3949)
  line L566 (66.2832, 13.3949) -> (67.2283, 13.1289)
  line L567 (67.2283, 13.1289) -> (67.544, 13.1289)
  line L568 (67.544, 13.1289) -> (67.8636, 13.1289)
  line L569 (67.8636, 13.1289) -> (68.8227, 13.2861)
  line L570 (68.8227, 13.2861) -> (69.6233, 13.6484)
  line L571 (69.6233, 13.6484) -> (69.7488, 13.7518)
  line L572 (69.7488, 13.7518) -> (69.8727, 13.8565)
  line L573 (69.8727, 13.8565) -> (70.3856, 14.5841)
  line L574 (70.3856, 14.5841) -> (70.7508, 15.59)
  line L575 (70.7508, 15.59) -> (70.8029, 15.8326)
  line L576 (74.3161, 11.4116) -> (74.3161, 16.2898)
  line L577 (74.3161, 16.2898) -> (76.1683, 16.2898)
  line L578 (76.1683, 16.2898) -> (76.2274, 16.0183)
  line L579 (76.2274, 16.0183) -> (76.6973, 14.8511)
  line L580 (76.6973, 14.8511) -> (77.3948, 13.9402)
  line L581 (77.3948, 13.9402) -> (77.5698, 13.7956)
  line L582 (77.5698, 13.7956) -> (77.7433, 13.6522)
  line L583 (77.7433, 13.6522) -> (78.7466, 13.1479)
  line L584 (78.7466, 13.1479) -> (79.8312, 12.9301)
  line L585 (79.8312, 12.9301) -> (80.1934, 12.9301)
  line L586 (80.1934, 12.9301) -> (80.41, 12.9301)
  line L587 (80.41, 12.9301) -> (81.0603, 13.0376)
  line L588 (81.0603, 13.0376) -> (81.6392, 13.2871)
  line L589 (81.6392, 13.2871) -> (81.7369, 13.3573)
  line L590 (81.7369, 13.3573) -> (81.8335, 13.429)
  line L591 (81.8335, 13.429) -> (82.171, 13.8562)
  line L592 (82.171, 13.8562) -> (82.3171, 14.3385)
  line L593 (82.3171, 14.3385) -> (82.3171, 14.4983)
  line L594 (82.3171, 14.4983) -> (82.3171, 14.7285)
  line L595 (82.3171, 14.7285) -> (81.9257, 15.361)
  line L596 (81.9257, 15.361) -> (81.8487, 15.4189)
  line L597 (81.8487, 15.4189) -> (81.77, 15.4781)
  line L598 (81.77, 15.4781) -> (81.1995, 15.7579)
  line L599 (81.1995, 15.7579) -> (80.3907, 16.0183)
  line L600 (80.3907, 16.0183) -> (80.1934, 16.0666)
  line L601 (80.1934, 16.0666) -> (78.3166, 16.5117)
  line L602 (78.3166, 16.5117) -> (77.9887, 16.593)
  line L603 (77.9887, 16.593) -> (76.6064, 17.1001)
  line L604 (76.6064, 17.1001) -> (75.5617, 17.7505)
  line L605 (75.5617, 17.7505) -> (75.4035, 17.9007)
  line L606 (75.4035, 17.9007) -> (75.245, 18.0523)
  line L607 (75.245, 18.0523) -> (74.6897, 18.9301)
  line L608 (74.6897, 18.9301) -> (74.4527, 19.8851)
  line L609 (74.4527, 19.8851) -> (74.4527, 20.2034)
  line L610 (74.4527, 20.2034) -> (74.4527, 20.5838)
  line L611 (74.4527, 20.5838) -> (74.7695, 21.722)
  line L612 (74.7695, 21.722) -> (75.5124, 22.7473)
  line L613 (75.5124, 22.7473) -> (75.7245, 22.9195)
  line L614 (75.7245, 22.9195) -> (75.9353, 23.0931)
  line L615 (75.9353, 23.0931) -> (77.199, 23.6981)
  line L616 (77.199, 23.6981) -> (78.6115, 23.9558)
  line L617 (78.6115, 23.9558) -> (79.0829, 23.9558)
  line L618 (79.0829, 23.9558) -> (79.5513, 23.9558)
  line L619 (79.5513, 23.9558) -> (80.8109, 23.705)
  line L620 (80.8109, 23.705) -> (80.9597, 23.654)
  line L621 (80.9597, 23.654) -> (81.107, 23.6044)
  line L622 (81.107, 23.6044) -> (82.5472, 22.8369)
  line L623 (82.5472, 22.8369) -> (82.6879, 22.7335)
  line L624 (82.6879, 22.7335) -> (83.2432, 23.672)
  line L625 (83.2432, 23.672) -> (84.6895, 23.672)
  line L626 (84.6895, 23.672) -> (84.6895, 19.2527)
  line L627 (84.6895, 19.2527) -> (82.9719, 19.2527)
  line L628 (82.9719, 19.2527) -> (82.9073, 19.4815)
  line L629 (82.9073, 19.4815) -> (82.4402, 20.4723)
  line L630 (82.4402, 20.4723) -> (81.7758, 21.2619)
  line L631 (81.7758, 21.2619) -> (81.6147, 21.3887)
  line L632 (81.6147, 21.3887) -> (81.4519, 21.5168)
  line L633 (81.4519, 21.5168) -> (80.5426, 21.9633)
  line L634 (80.5426, 21.9633) -> (79.5957, 22.1548)
  line L635 (79.5957, 22.1548) -> (79.28, 22.1548)
  line L636 (79.28, 22.1548) -> (79.0788, 22.1548)
  line L637 (79.0788, 22.1548) -> (78.4753, 22.0611)
  line L638 (78.4753, 22.0611) -> (77.9518, 21.8407)
  line L639 (77.9518, 21.8407) -> (77.8665, 21.7773)
  line L640 (77.8665, 21.7773) -> (77.7806, 21.7152)
  line L641 (77.7806, 21.7152) -> (77.4819, 21.3294)
  line L642 (77.4819, 21.3294) -> (77.3549, 20.8829)
  line L643 (77.3549, 20.8829) -> (77.3549, 20.7341)
  line L644 (77.3549, 20.7341) -> (77.3549, 20.5356)
  line L645 (77.3549, 20.5356) -> (77.6432, 19.9899)
  line L646 (77.6432, 19.9899) -> (77.7008, 19.9376)
  line L647 (77.7008, 19.9376) -> (77.7575, 19.8852)
  line L648 (77.7575, 19.8852) -> (78.653, 19.4786)
  line L649 (78.653, 19.4786) -> (78.7744, 19.4496)
  line L650 (78.7744, 19.4496) -> (81.0716, 18.9189)
  line L651 (81.0716, 18.9189) -> (81.4406, 18.8307)
  line L652 (81.4406, 18.8307) -> (82.9897, 18.2862)
  line L653 (82.9897, 18.2862) -> (84.136, 17.6068)
  line L654 (84.136, 17.6068) -> (84.3059, 17.4496)
  line L655 (84.3059, 17.4496) -> (84.4738, 17.2939)
  line L656 (84.4738, 17.2939) -> (85.0648, 16.3706)
  line L657 (85.0648, 16.3706) -> (85.3186, 15.3467)
  line L658 (85.3186, 15.3467) -> (85.3186, 15.005)
  line L659 (85.3186, 15.005) -> (85.3186, 14.6026)
  line L660 (85.3186, 14.6026) -> (84.9962, 13.3941)
  line L661 (84.9962, 13.3941) -> (84.248, 12.3385)
  line L662 (84.248, 12.3385) -> (84.0341, 12.1648)
  line L663 (84.0341, 12.1648) -> (83.8192, 11.9926)
  line L664 (83.8192, 11.9926) -> (82.5045, 11.3876)
  line L665 (82.5045, 11.3876) -> (80.9927, 11.1272)
  line L666 (80.9927, 11.1272) -> (80.4898, 11.1272)
  line L667 (80.4898, 11.1272) -> (79.9703, 11.1272)
  line L668 (79.9703, 11.1272) -> (78.5741, 11.3906)
  line L669 (78.5741, 11.3906) -> (78.4159, 11.4429)
  line L670 (78.4159, 11.4429) -> (78.2574, 11.4953)
  line L671 (78.2574, 11.4953) -> (76.6218, 12.3554)
  line L672 (76.6218, 12.3554) -> (76.4539, 12.474)
  line L673 (76.4539, 12.474) -> (75.996, 11.4116)
  line L674 (75.996, 11.4116) -> (74.3161, 11.4116)
  line L675 (86.4817, 11.4116) -> (86.4817, 16.2898)
  line L676 (86.4817, 16.2898) -> (88.3338, 16.2898)
  line L677 (88.3338, 16.2898) -> (88.393, 16.0183)
  line L678 (88.393, 16.0183) -> (88.8629, 14.8511)
  line L679 (88.8629, 14.8511) -> (89.5601, 13.9402)
  line L680 (89.5601, 13.9402) -> (89.7352, 13.7956)
  line L681 (89.7352, 13.7956) -> (89.9086, 13.6522)
  line L682 (89.9086, 13.6522) -> (90.9119, 13.1479)
  line L683 (90.9119, 13.1479) -> (91.9963, 12.9302)
  line L684 (91.9963, 12.9302) -> (92.359, 12.9302)
  line L685 (92.359, 12.9302) -> (92.5751, 12.9302)
  line L686 (92.5751, 12.9302) -> (93.2259, 13.0377)
  line L687 (93.2259, 13.0377) -> (93.8042, 13.2871)
  line L688 (93.8042, 13.2871) -> (93.9023, 13.3574)
  line L689 (93.9023, 13.3574) -> (93.9988, 13.429)
  line L690 (93.9988, 13.429) -> (94.3364, 13.8562)
  line L691 (94.3364, 13.8562) -> (94.4824, 14.3385)
  line L692 (94.4824, 14.3385) -> (94.4824, 14.4984)
  line L693 (94.4824, 14.4984) -> (94.4824, 14.7285)
  line L694 (94.4824, 14.7285) -> (94.0897, 15.3611)
  line L695 (94.0897, 15.3611) -> (94.0125, 15.4189)
  line L696 (94.0125, 15.4189) -> (93.934, 15.4782)
  line L697 (93.934, 15.4782) -> (93.3633, 15.7579)
  line L698 (93.3633, 15.7579) -> (92.5558, 16.0184)
  line L699 (92.5558, 16.0184) -> (92.359, 16.0666)
  line L700 (92.359, 16.0666) -> (90.4819, 16.5118)
  line L701 (90.4819, 16.5118) -> (90.154, 16.5931)
  line L702 (90.154, 16.5931) -> (88.7705, 17.1002)
  line L703 (88.7705, 17.1002) -> (87.726, 17.7506)
  line L704 (87.726, 17.7506) -> (87.5675, 17.9008)
  line L705 (87.5675, 17.9008) -> (87.4088, 18.0524)
  line L706 (87.4088, 18.0524) -> (86.8535, 18.9302)
  line L707 (86.8535, 18.9302) -> (86.6166, 19.8852)
  line L708 (86.6166, 19.8852) -> (86.6166, 20.2035)
  line L709 (86.6166, 20.2035) -> (86.6166, 20.5839)
  line L710 (86.6166, 20.5839) -> (86.9336, 21.7221)
  line L711 (86.9336, 21.7221) -> (87.6763, 22.7474)
  line L712 (87.6763, 22.7474) -> (87.8886, 22.9196)
  line L713 (87.8886, 22.9196) -> (88.0992, 23.0932)
  line L714 (88.0992, 23.0932) -> (89.3633, 23.6982)
  line L715 (89.3633, 23.6982) -> (90.7753, 23.9558)
  line L716 (90.7753, 23.9558) -> (91.2468, 23.9558)
  line L717 (91.2468, 23.9558) -> (91.7151, 23.9558)
  line L718 (91.7151, 23.9558) -> (92.975, 23.705)
  line L719 (92.975, 23.705) -> (93.1238, 23.654)
  line L720 (93.1238, 23.654) -> (93.2714, 23.6044)
  line L721 (93.2714, 23.6044) -> (94.7114, 22.8369)
  line L722 (94.7114, 22.8369) -> (94.8518, 22.7335)
  line L723 (94.8518, 22.7335) -> (95.4085, 23.6721)
  line L724 (95.4085, 23.6721) -> (96.8531, 23.6721)
  line L725 (96.8531, 23.6721) -> (96.8531, 19.2527)
  line L726 (96.8531, 19.2527) -> (95.1376, 19.2527)
  line L727 (95.1376, 19.2527) -> (95.0726, 19.4815)
  line L728 (95.0726, 19.4815) -> (94.6055, 20.4723)
  line L729 (94.6055, 20.4723) -> (93.9413, 21.2619)
  line L730 (93.9413, 21.2619) -> (93.7787, 21.3887)
  line L731 (93.7787, 21.3887) -> (93.6159, 21.5168)
  line L732 (93.6159, 21.5168) -> (92.7066, 21.9633)
  line L733 (92.7066, 21.9633) -> (91.7597, 22.1548)
  line L734 (91.7597, 22.1548) -> (91.4457, 22.1548)
  line L735 (91.4457, 22.1548) -> (91.2445, 22.1548)
  line L736 (91.2445, 22.1548) -> (90.641, 22.0611)
  line L737 (90.641, 22.0611) -> (90.117, 21.8407)
  line L738 (90.117, 21.8407) -> (90.0317, 21.7773)
  line L739 (90.0317, 21.7773) -> (89.9464, 21.7152)
  line L740 (89.9464, 21.7152) -> (89.6471, 21.3294)
  line L741 (89.6471, 21.3294) -> (89.5191, 20.8829)
  line L742 (89.5191, 20.8829) -> (89.5191, 20.7341)
  line L743 (89.5191, 20.7341) -> (89.5191, 20.5356)
  line L744 (89.5191, 20.5356) -> (89.8069, 19.99)
  line L745 (89.8069, 19.99) -> (89.8648, 19.9376)
  line L746 (89.8648, 19.9376) -> (89.9217, 19.8852)
  line L747 (89.9217, 19.8852) -> (90.8173, 19.4786)
  line L748 (90.8173, 19.4786) -> (90.9384, 19.4496)
  line L749 (90.9384, 19.4496) -> (93.2356, 18.9189)
  line L750 (93.2356, 18.9189) -> (93.6049, 18.8307)
  line L751 (93.6049, 18.8307) -> (95.154, 18.2862)
  line L752 (95.154, 18.2862) -> (96.3004, 17.6066)
  line L753 (96.3004, 17.6066) -> (96.4695, 17.4495)
  line L754 (96.4695, 17.4495) -> (96.6379, 17.2938)
  line L755 (96.6379, 17.2938) -> (97.2287, 16.3705)
  line L756 (97.2287, 16.3705) -> (97.4825, 15.3466)
  line L757 (97.4825, 15.3466) -> (97.4825, 15.0049)
  line L758 (97.4825, 15.0049) -> (97.4825, 14.6025)
  line L759 (97.4825, 14.6025) -> (97.1599, 13.3939)
  line L760 (97.1599, 13.3939) -> (96.4118, 12.3384)
  line L761 (96.4118, 12.3384) -> (96.1982, 12.1648)
  line L762 (96.1982, 12.1648) -> (95.983, 11.9925)
  line L763 (95.983, 11.9925) -> (94.6696, 11.3876)
  line L764 (94.6696, 11.3876) -> (93.158, 11.1272)
  line L765 (93.158, 11.1272) -> (92.6554, 11.1272)
  line L766 (92.6554, 11.1272) -> (92.1357, 11.1272)
  line L767 (92.1357, 11.1272) -> (90.7384, 11.3906)
  line L768 (90.7384, 11.3906) -> (90.5812, 11.4429)
  line L769 (90.5812, 11.4429) -> (90.4225, 11.4953)
  line L770 (90.4225, 11.4953) -> (88.7858, 12.3554)
  line L771 (88.7858, 12.3554) -> (88.6177, 12.474)
  line L772 (88.6177, 12.474) -> (88.1598, 11.4116)
  line L773 (88.1598, 11.4116) -> (86.4817, 11.4116)
  line L774 (107.1895, 19.0679) -> (107.1698, 19.3435)
  line L775 (107.1698, 19.3435) -> (106.966, 20.4997)
  line L776 (106.966, 20.4997) -> (106.6104, 21.3596)
  line L777 (106.6104, 21.3596) -> (106.5169, 21.4864)
  line L778 (106.5169, 21.4864) -> (106.4232, 21.6145)
  line L779 (106.4232, 21.6145) -> (105.8225, 22.0624)
  line L780 (105.8225, 22.0624) -> (105.107, 22.2526)
  line L781 (105.107, 22.2526) -> (104.8687, 22.2526)
  line L782 (104.8687, 22.2526) -> (104.6165, 22.2526)
  line L783 (104.6165, 22.2526) -> (103.8599, 22.0513)
  line L784 (103.8599, 22.0513) -> (103.1751, 21.5787)
  line L785 (103.1751, 21.5787) -> (103.0595, 21.4437)
  line L786 (103.0595, 21.4437) -> (102.9424, 21.31)
  line L787 (102.9424, 21.31) -> (102.4806, 20.4459)
  line L788 (102.4806, 20.4459) -> (102.1761, 19.3298)
  line L789 (102.1761, 19.3298) -> (102.14, 19.0679)
  line L790 (102.14, 19.0679) -> (107.1895, 19.0679)
  line L791 (108.3384, 15.8331) -> (110.4615, 15.8331)
  line L792 (110.4615, 15.8331) -> (110.4161, 15.4679)
  line L793 (110.4161, 15.4679) -> (109.8857, 13.8693)
  line L794 (109.8857, 13.8693) -> (108.9504, 12.5808)
  line L795 (108.9504, 12.5808) -> (108.7023, 12.3698)
  line L796 (108.7023, 12.3698) -> (108.4544, 12.159)
  line L797 (108.4544, 12.159) -> (107.006, 11.4214)
  line L798 (107.006, 11.4214) -> (105.4214, 11.1042)
  line L799 (105.4214, 11.1042) -> (104.8938, 11.1042)
  line L800 (104.8938, 11.1042) -> (104.5504, 11.1042)
  line L801 (104.5504, 11.1042) -> (103.5212, 11.2145)
  line L802 (103.5212, 11.2145) -> (102.2977, 11.5411)
  line L803 (102.2977, 11.5411) -> (101.2185, 12.087)
  line L804 (101.2185, 12.087) -> (100.4979, 12.6381)
  line L805 (100.4979, 12.6381) -> (100.2883, 12.8503)
  line L806 (100.2883, 12.8503) -> (100.0777, 13.0653)
  line L807 (100.0777, 13.0653) -> (99.5356, 13.7984)
  line L808 (99.5356, 13.7984) -> (98.9996, 14.8925)
  line L809 (98.9996, 14.8925) -> (98.6772, 16.1354)
  line L810 (98.6772, 16.1354) -> (98.5711, 17.1772)
  line L811 (98.5711, 17.1772) -> (98.5711, 17.5245)
  line L812 (98.5711, 17.5245) -> (98.5711, 17.869)
  line L813 (98.5711, 17.869) -> (98.6787, 18.8998)
  line L814 (98.6787, 18.8998) -> (99.004, 20.1345)
  line L815 (99.004, 20.1345) -> (99.5471, 21.23)
  line L816 (99.5471, 21.23) -> (100.0938, 21.9686)
  line L817 (100.0938, 21.9686) -> (100.3064, 22.1849)
  line L818 (100.3064, 22.1849) -> (100.5172, 22.4013)
  line L819 (100.5172, 22.4013) -> (101.2431, 22.9607)
  line L820 (101.2431, 22.9607) -> (102.3196, 23.5133)
  line L821 (102.3196, 23.5133) -> (103.5362, 23.8455)
  line L822 (103.5362, 23.8455) -> (104.5533, 23.9557)
  line L823 (104.5533, 23.9557) -> (104.8939, 23.9557)
  line L824 (104.8939, 23.9557) -> (105.2162, 23.9557)
  line L825 (105.2162, 23.9557) -> (106.1877, 23.8496)
  line L826 (106.1877, 23.8496) -> (107.3191, 23.5299)
  line L827 (107.3191, 23.5299) -> (108.2866, 22.9952)
  line L828 (108.2866, 22.9952) -> (108.9147, 22.455)
  line L829 (108.9147, 22.455) -> (109.0912, 22.2469)
  line L830 (109.0912, 22.2469) -> (109.2731, 22.0306)
  line L831 (109.2731, 22.0306) -> (109.7222, 21.2947)
  line L832 (109.7222, 21.2947) -> (110.1745, 20.1496)
  line L833 (110.1745, 20.1496) -> (110.4442, 18.8101)
  line L834 (110.4442, 18.8101) -> (110.5351, 17.6617)
  line L835 (110.5351, 17.6617) -> (110.5351, 17.2775)
  line L836 (110.5351, 17.2775) -> (102.016, 17.2775)
  line L837 (102.016, 17.2775) -> (102.0281, 16.9412)
  line L838 (102.0281, 16.9412) -> (102.2666, 15.4943)
  line L839 (102.2666, 15.4943) -> (102.7433, 14.3684)
  line L840 (102.7433, 14.3684) -> (102.8741, 14.1906)
  line L841 (102.8741, 14.1906) -> (103.0036, 14.0142)
  line L842 (103.0036, 14.0142) -> (103.8166, 13.3954)
  line L843 (103.8166, 13.3954) -> (104.762, 13.1294)
  line L844 (104.762, 13.1294) -> (105.0775, 13.1294)
  line L845 (105.0775, 13.1294) -> (105.3975, 13.1294)
  line L846 (105.3975, 13.1294) -> (106.3564, 13.2865)
  line L847 (106.3564, 13.2865) -> (107.1573, 13.6489)
  line L848 (107.1573, 13.6489) -> (107.2825, 13.7523)
  line L849 (107.2825, 13.7523) -> (107.4067, 13.857)
  line L850 (107.4067, 13.857) -> (107.9193, 14.5846)
  line L851 (107.9193, 14.5846) -> (108.2858, 15.5906)
  line L852 (108.2858, 15.5906) -> (108.3384, 15.8331)
  line L853 (120.395, 19.0679) -> (120.3759, 19.3434)
  line L854 (120.3759, 19.3434) -> (120.1704, 20.4997)
  line L855 (120.1704, 20.4997) -> (119.8149, 21.3596)
  line L856 (119.8149, 21.3596) -> (119.7212, 21.4864)
  line L857 (119.7212, 21.4864) -> (119.6277, 21.6145)
  line L858 (119.6277, 21.6145) -> (119.028, 22.0624)
  line L859 (119.028, 22.0624) -> (118.3115, 22.2525)
  line L860 (118.3115, 22.2525) -> (118.0729, 22.2525)
  line L861 (118.0729, 22.2525) -> (117.8207, 22.2525)
  line L862 (117.8207, 22.2525) -> (117.0643, 22.0513)
  line L863 (117.0643, 22.0513) -> (116.3795, 21.5787)
  line L864 (116.3795, 21.5787) -> (116.2637, 21.4437)
  line L865 (116.2637, 21.4437) -> (116.1463, 21.31)
  line L866 (116.1463, 21.31) -> (115.6851, 20.4459)
  line L867 (115.6851, 20.4459) -> (115.3815, 19.3298)
  line L868 (115.3815, 19.3298) -> (115.3447, 19.0679)
  line L869 (115.3447, 19.0679) -> (120.395, 19.0679)
  line L870 (121.5423, 15.8329) -> (123.666, 15.8329)
  line L871 (123.666, 15.8329) -> (123.6206, 15.4678)
  line L872 (123.6206, 15.4678) -> (123.0902, 13.8692)
  line L873 (123.0902, 13.8692) -> (122.1549, 12.5806)
  line L874 (122.1549, 12.5806) -> (121.907, 12.3697)
  line L875 (121.907, 12.3697) -> (121.6586, 12.1588)
  line L876 (121.6586, 12.1588) -> (120.2104, 11.4213)
  line L877 (120.2104, 11.4213) -> (118.626, 11.1042)
  line L878 (118.626, 11.1042) -> (118.0982, 11.1042)
  line L879 (118.0982, 11.1042) -> (117.7548, 11.1042)
  line L880 (117.7548, 11.1042) -> (116.7256, 11.2145)
  line L881 (116.7256, 11.2145) -> (115.5018, 11.5412)
  line L882 (115.5018, 11.5412) -> (114.4228, 12.0869)
  line L883 (114.4228, 12.0869) -> (113.7022, 12.638)
  line L884 (113.7022, 12.638) -> (113.4926, 12.8503)
  line L885 (113.4926, 12.8503) -> (113.2816, 13.0653)
  line L886 (113.2816, 13.0653) -> (112.7415, 13.7983)
  line L887 (112.7415, 13.7983) -> (112.2055, 14.8925)
  line L888 (112.2055, 14.8925) -> (111.8827, 16.1355)
  line L889 (111.8827, 16.1355) -> (111.777, 17.1772)
  line L890 (111.777, 17.1772) -> (111.777, 17.5245)
  line L891 (111.777, 17.5245) -> (111.777, 17.869)
  line L892 (111.777, 17.869) -> (111.8842, 18.8998)
  line L893 (111.8842, 18.8998) -> (112.2094, 20.1345)
  line L894 (112.2094, 20.1345) -> (112.751, 21.23)
  line L895 (112.751, 21.23) -> (113.2996, 21.9686)
  line L896 (113.2996, 21.9686) -> (113.512, 22.185)
  line L897 (113.512, 22.185) -> (113.7225, 22.4013)
  line L898 (113.7225, 22.4013) -> (114.4477, 22.9608)
  line L899 (114.4477, 22.9608) -> (115.5254, 23.5134)
  line L900 (115.5254, 23.5134) -> (116.7406, 23.8455)
  line L901 (116.7406, 23.8455) -> (117.7576, 23.9557)
  line L902 (117.7576, 23.9557) -> (118.0982, 23.9557)
  line L903 (118.0982, 23.9557) -> (118.4205, 23.9557)
  line L904 (118.4205, 23.9557) -> (119.3921, 23.8496)
  line L905 (119.3921, 23.8496) -> (120.5234, 23.5299)
  line L906 (120.5234, 23.5299) -> (121.4909, 22.9952)
  line L907 (121.4909, 22.9952) -> (122.119, 22.455)
  line L908 (122.119, 22.455) -> (122.2956, 22.247)
  line L909 (122.2956, 22.247) -> (122.4774, 22.0306)
  line L910 (122.4774, 22.0306) -> (122.9268, 21.2947)
  line L911 (122.9268, 21.2947) -> (123.3786, 20.1496)
  line L912 (123.3786, 20.1496) -> (123.6501, 18.8101)
  line L913 (123.6501, 18.8101) -> (123.7405, 17.6608)
  line L914 (123.7405, 17.6608) -> (123.7405, 17.2772)
  line L915 (123.7405, 17.2772) -> (115.2202, 17.2772)
  line L916 (115.2202, 17.2772) -> (115.2329, 16.941)
  line L917 (115.2329, 16.941) -> (115.4708, 15.494)
  line L918 (115.4708, 15.494) -> (115.9478, 14.3682)
  line L919 (115.9478, 14.3682) -> (116.0786, 14.1904)
  line L920 (116.0786, 14.1904) -> (116.2081, 14.014)
  line L921 (116.2081, 14.014) -> (117.0211, 13.3952)
  line L922 (117.0211, 13.3952) -> (117.9665, 13.1292)
  line L923 (117.9665, 13.1292) -> (118.282, 13.1292)
  line L924 (118.282, 13.1292) -> (118.6017, 13.1292)
  line L925 (118.6017, 13.1292) -> (119.5609, 13.2863)
  line L926 (119.5609, 13.2863) -> (120.3617, 13.6487)
  line L927 (120.3617, 13.6487) -> (120.4869, 13.7521)
  line L928 (120.4869, 13.7521) -> (120.6111, 13.8568)
  line L929 (120.6111, 13.8568) -> (121.1237, 14.5844)
  line L930 (121.1237, 14.5844) -> (121.4902, 15.5904)
  line L931 (121.4902, 15.5904) -> (121.5423, 15.8329)
  line L932 (45.6766, 7.5792) -> (45.514, 7.5792)
  line L933 (45.514, 7.5792) -> (45.3001, 7.5792)
  line L934 (45.3001, 7.5792) -> (44.6596, 7.4318)
  line L935 (44.6596, 7.4318) -> (44.1495, 7.0872)
  line L936 (44.1495, 7.0872) -> (44.0754, 6.988)